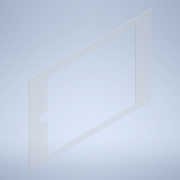
# Autodesk Inventor part: lc_box_side
Saved by Autodesk Inventor 2021.1 (Build 251245010, 245A)
## iProperties
Created: 2019-07-19
Part Number: lc_box_side
Material: ポリカーボネート、クリア
Document SubType Name: Modeling
Designer: gisen
Density: 1.2 g/cm^3
Appearance: ポリカーボネート - クリア
Mass: 185.38 g
Surface Area: 1454.08 cm^2
Volume: 185.38 cm^3
Author: gisen
Autodesk Inventor part; units mm, degrees
ref_plane "YZ Plane" through (0, 0, 0) normal (1, 0, 0) x (0, 1, 0)
ref_plane "XZ Plane" through (0, 0, 0) normal (0, 1, 0) x (-1, 0, 0)
ref_plane "XY Plane" through (0, 0, 0) normal (0, 0, 1) x (1, 0, 0)
sketch "スケッチ1" plane through (0, 0, 0) normal (1, 0, 0) x (0, 1, 0)
  line L0 (125.6523, 179.1954) -> (-64.3477, 179.1954)
  line L1 (-64.3477, 179.1954) -> (-64.3477, -110.8046)
  line L2 (-64.3477, -110.8046) -> (125.6523, -110.8046)
  line L3 (125.6523, -110.8046) -> (125.6523, 179.1954)
  point P0 (0, 0)
  dimension "d0" = 190
  dimension "d1" = 290
  constraints: 8 end point, 2 parallel, 1 horizontal, 1 perpendicular
  measures "d0" distance of L0.start L0.end
  measures "d1" distance of L2.end L0.start
extrude "押し出し1" add sketch "スケッチ1" along normal blind 2.6
sketch "スケッチ2" plane through (2.6, 0, 0) normal (1, 0, 0) x (0, 0, -1)
  line L0 (-179.1954, 125.6523) -> (-179.1954, -64.3477) projected
  line L1 (-179.1954, -64.3477) -> (110.8046, -64.3477) projected
  line L2 (110.8046, -64.3477) -> (110.8046, 125.6523) projected
  line L3 (110.8046, 125.6523) -> (-179.1954, 125.6523) projected
  line L4 (-34.1954, 30.6523) -> (-34.1954, 125.6523)
  line L5 (110.8046, 125.6523) -> (-179.1954, 125.6523) projected
  line L6 (-34.1954, 30.6523) -> (110.8046, 30.6523)
  point P0 (0, 0)
  point P1 (-169.1954, 115.6523)
  point P2 (100.8046, 115.6523)
  point P3 (-169.1954, -54.3477)
  point P4 (100.8046, -54.3477)
  dimension "d4" = 10
  dimension "d5" = 10
  constraints: 4 end point, 3 symmetric about line, 2 midpoint
  measures "d4" distance from line of L3 point (-169.195, 115.652)
  measures "d5" distance from line of L0 point (-169.195, 115.652)
hole "穴1" at (2.6, 115.6523, 169.1954) at (2.6, 115.6523, -100.8046) at (2.6, -54.3477, 169.1954) at (2.6, -54.3477, -100.8046) direction (-1, 0, 0) diameter 4.5 depth 10 tip angle 118
sketch "スケッチ4" plane through (0, 0, 0) normal (-1, 0, 0) x (0, 0, 1)
  line L0 (-73.8046, -50.3477) -> (-73.8046, 108.6523) projected
  line L1 (-73.8046, 108.6523) -> (136.1954, 108.6523) projected
  line L2 (136.1954, 108.6523) -> (136.1954, -50.3477) projected
  line L3 (136.1954, -50.3477) -> (-73.8046, -50.3477) projected
  point P0 (0, 0)
extrude "押し出し3" cut sketch "スケッチ4" against normal blind 10
sketch "スケッチ5" plane through (0, 0, 0) normal (-1, 0, 0) x (0, 0, 1)
  circle A0 centre (146.6954, 29.1523) radius 5.5 projected
  line L0 (136.1954, 108.6523) -> (136.1954, -50.3477) projected
  line L1 (136.1954, 37.6523) -> (154.6954, 37.6523)
  line L2 (154.6954, 37.6523) -> (154.6954, 20.6523)
  line L3 (154.6954, 20.6523) -> (136.1954, 20.6523)
  line L4 (136.1954, 20.6523) -> (136.1954, 37.6523)
  point P0 (0, 0)
  point P1 (136.1954, 20.6523)
  dimension "d21" = 8
  dimension "d22" = 8.5
  dimension "d23" = 8.5
  constraints: 8 end point, 2 parallel, 1 horizontal, 1 perpendicular, 1 point on line
  measures "d21" distance from line of L2 A0.centre
  measures "d22" distance from line of L3 A0.centre
  measures "d23" distance from line of A0.centre L1
extrude "押し出し4" cut sketch "スケッチ5" against normal blind 10 contours A0 | L1 L2 L3 L0
fillet "フィレット1" radius 8 4 edges at (1.3, 37.6523, 154.6954) (1.3, 20.6523, 154.6954) (1.3, 37.6523, 136.1954) (1.3, 20.6523, 136.1954)
